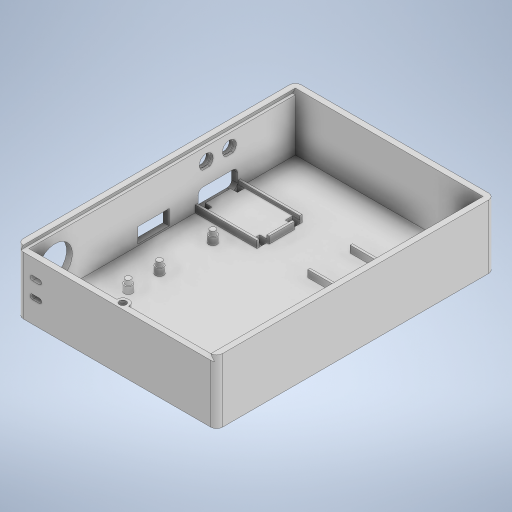
# Autodesk Inventor part: 01-Electronic-Compartment-Updated
Saved by Autodesk Inventor 2023 (Build 270158000, 158)
## iProperties
Created: 2024-02-14
Part Number: 01-Electronic-Compartment-Updated
Material: Generic
Document SubType Name: Modeling
Designer: ongyu
Density: 1 g/cm^3
Appearance: Default
Author: ongyu
Autodesk Inventor part; units mm, degrees
ref_plane "YZ Plane" through (0, 0, 0) normal (1, 0, 0) x (0, 1, 0)
ref_plane "XZ Plane" through (0, 0, 0) normal (0, 1, 0) x (-1, 0, 0)
sketch "Sketch1" plane through (0, 0, 0) normal (0, 1, 0) x (-1, 0, 0)
  line L0 (38, -43.8749) -> (-38, -43.8749)
  line L1 (-38, -43.8749) -> (-38, -23.8749)
  line L2 (-38, -23.8749) -> (38, -23.8749)
  line L3 (38, -23.8749) -> (38, -43.8749)
  line L4 (0, -70.3716) -> (0, 97.6051) projected
  line L5 (43, -43.8749) -> (-38, -43.8749)
  line L6 (-38, -43.8749) -> (-38, 71.1084)
  line L7 (-38, 71.1084) -> (43, 71.1084)
  line L8 (43, 71.1084) -> (43, -43.8749)
  circle A0 centre (-29.9129, 6.6001) radius 1.275
  circle A1 centre (-29.9129, 29.6501) radius 1.275
  circle A2 centre (28.1371, 6.6001) radius 1.275
  circle A3 centre (28.1371, 29.6501) radius 1.275
  line L9 (45.5, -46.3749) -> (-40.5, -46.3749)
  line L10 (-40.5, -46.3749) -> (-40.5, 73.6084)
  line L11 (-40.5, 73.6084) -> (45.5, 73.6084)
  line L12 (45.5, 73.6084) -> (45.5, -46.3749)
  line L13 (43, -18.8749) -> (14.338, -18.8749)
  line L14 (43, -1.8749) -> (14.338, -1.8749)
  line L15 (43, -18.8749) -> (40, -18.8749)
  line L16 (40, -18.8749) -> (40, -15.8749)
  line L17 (40, -15.8749) -> (43, -15.8749)
  line L18 (43, -15.8749) -> (43, -18.8749)
  line L19 (43, -1.8749) -> (40, -1.8749)
  line L20 (40, -1.8749) -> (40, -4.8749)
  line L21 (40, -4.8749) -> (43, -4.8749)
  line L22 (43, -4.8749) -> (43, -1.8749)
  line L23 (19.338, -1.8749) -> (16.338, -1.8749)
  line L24 (16.338, -1.8749) -> (16.338, -4.8749)
  line L25 (16.338, -4.8749) -> (19.338, -4.8749)
  line L26 (19.338, -4.8749) -> (19.338, -1.8749)
  line L27 (19.338, -18.8749) -> (16.338, -18.8749)
  line L28 (16.338, -18.8749) -> (16.338, -15.8749)
  line L29 (16.338, -15.8749) -> (19.338, -15.8749)
  line L30 (19.338, -15.8749) -> (19.338, -18.8749)
  line L31 (32, 3.1251) -> (-33, 3.1251)
  line L32 (-33, 3.1251) -> (-33, 33.1251)
  line L33 (-33, 33.1251) -> (32, 33.1251)
  line L34 (32, 33.1251) -> (32, 3.1251)
  line L35 (32, 18.1251) -> (-33, 18.1251)
  point P0 (0, 0)
  point P1 (43, -4.8749)
  point P2 (43, -15.8749)
  dimension "d0" = 76
  dimension "d1" = 20
  dimension "d2" = 38
  dimension "d4" = 5
  dimension "d5" = 0
  dimension "d14" = 2.55
  dimension "d15" = 2.55
  dimension "d17" = 2.55
  dimension "d18" = 58.05
  dimension "d24" = 81
  dimension "d31" = 0
  dimension "d32" = 2.5
  dimension "d33" = 2.5
  dimension "d34" = 2.5
  dimension "d35" = 2.5
  dimension "d72" = 17
  dimension "d73" = 28.662
  dimension "d74" = 28.662
  dimension "d75" = 3
  dimension "d76" = 3
  dimension "d77" = 3
  dimension "d78" = 3
  dimension "d79" = 2
  dimension "d80" = 3
  dimension "d81" = 3
  dimension "d82" = 3
  dimension "d83" = 3
  dimension "d115" = 65
  dimension "d116" = 30
  dimension "d119" = 5
  dimension "d120" = 5
  dimension "d209" = 114.9833
  dimension "d210" = 119.9833
  dimension "d268" = 5
  dimension "d270" = 3.0871
  dimension "d273" = 0
  dimension "d274" = 0
  dimension "d275" = 23.05
  dimension "d276" = 23.05
  constraints: 70 end point, 16 parallel, 10 horizontal, 9 perpendicular, 4 centre point, 4 point on line, 2 midpoint
  measures "d0" distance of L0.start L0.end
  measures "d1" distance of L2.end L0.start
  measures "d2" distance between parallel lines of L4 L3
  measures "d4" distance between parallel lines of L8 L3
  measures "d5" distance between parallel lines of L6 L1
  measures "d14" diameter of A0
  measures "d15" diameter of A1
  measures "d17" diameter of A2
  measures "d18" distance of A2.centre A0.centre
  measures "d24" distance of L5.start L5.end
  measures "d31" distance between parallel lines of L5 L0
  measures "d32" distance between parallel lines of L11 L7
  measures "d33" distance between parallel lines of L10 L6
  measures "d34" distance between parallel lines of L12 L8
  measures "d35" distance between parallel lines of L0 L9
  measures "d72" distance between parallel lines of L14 L13
  measures "d73" distance of L13.start L13.end
  measures "d74" distance of L14.start L14.end
  measures "d75" distance of L15.end L16.end
  measures "d76" distance of L16.end L17.end
  measures "d77" distance of L20.end L21.end
  measures "d78" distance of L19.end L20.end
  measures "d79" distance from line of L14.end L24
  measures "d80" distance of L24.end L25.end
  measures "d81" distance of L25.end L23.start
  measures "d82" distance of L28.end L29.end
  measures "d83" distance of L29.end L27.start
  measures "d115" distance between parallel lines of L34 L32
  measures "d116" distance between parallel lines of L33 L31
  measures "d119" distance between parallel lines of L13 L2
  measures "d120" distance between parallel lines of L31 L14
  measures "d209" distance between parallel lines of L7 L0
  measures "d210" distance between parallel lines of L11 L9
  measures "d268" distance between parallel lines of L6 L32
  measures "d270" distance from line of L32 A0.centre
  measures "d273" horizontal distance of A1.centre A0.centre
  measures "d274" horizontal distance of A3.centre A2.centre
  measures "d275" distance of A1.centre A0.centre
  measures "d276" distance of A2.centre A3.centre
extrude "Extrusion3" add sketch "Sketch1" along normal blind 25 contours L5 L8 L7 L4 L11 L12 L9 L0 | L4 L9 L10 L11 L7 L6 L1 L0
extrude "Extrusion12" add sketch "Sketch1" against normal blind 2.5 contours L5 L8 L7 L4 L11 L12 L9 L0 | L0 L4 L2 L3 | L3 L2 L4 L31 L34 L33 L7 L8 L14 L20 L21 L17 L16 L13 L5 | L4 L9 L10 L11 L7 L6 L1 L0 | L0 L1 L2 L4 | L2 L6 L7 L4 L33 L32 L31 | L13 L16 L17 L8 | L31 L32 L35 L4 | L4 L35 L34 L31 | L35 L32 L33 L4 | L4 L33 L34 L35 | L21 L20 L14 L8 | A0 | A1 | A2 | A3 | L13 L28 L29 L30 | L26 L25 L24 L14
fillet "Fillet6" radius 2.5 4 edges at (40.5, 11.25, 73.6084) (-45.5, 11.25, 73.6084) (40.5, 11.25, -46.3749) (-45.5, 11.25, -46.3749)
extrude "Extrusion1" add sketch "Sketch1" along normal blind 5 contours A0 | A2 | A3
sketch "Sketch11" plane through (0, 0, 0) normal (0, 1, 0) x (1, 0, 0)
  circle A0 centre (-28.1371, -6.6001) radius 1.275 projected
  circle A1 centre (-28.1371, -29.6501) radius 1.275 projected
  circle A2 centre (29.9129, -6.6001) radius 1.275 projected
  circle A3 centre (-28.1371, -6.6001) radius 1.775
  circle A4 centre (-28.1371, -29.6501) radius 1.775
  circle A5 centre (29.9129, -6.6001) radius 1.775
  point P0 (0, 0)
  point P1 (26.525, -36.3729)
  dimension "d105" = 3.55
  dimension "d107" = 3.55
  dimension "d108" = 3.55
  dimension "d109" = 2.55
  constraints: 3 centre point, 3 coincident
  measures "d105" diameter of A5
  measures "d107" diameter of A4
  measures "d108" diameter of A3
  measures "d109" diameter of A2
extrude "Extrusion13" add sketch "Sketch11" along normal blind 3 contours A0 | A1 | A2 | A3 | A4 | A5
extrude "Extrusion14" cut sketch "Sketch1" against normal blind 2 contours L13 L16 L17 L8 | L21 L20 L14 L8 | L13 L28 L29 L30 | L26 L25 L24 L14
sketch "Sketch12" plane through (-45.5, -2.5, -43.8749) normal (-1, 0, 0) x (0, 0, 1)
  line L0 (25, 2.5) -> (25, 0.5) projected
  line L1 (27, 2.5) -> (40, 2.5)
  line L2 (42, 4.5) -> (42, 8.5)
  line L3 (40, 10.5) -> (27, 10.5)
  line L4 (25, 8.5) -> (25, 4.5)
  arc A0 (27, 10.5) -> (25, 8.5) centre (27, 8.5) ccw
  arc A1 (25, 4.5) -> (27, 2.5) centre (27, 4.5) ccw
  arc A2 (40, 2.5) -> (42, 4.5) centre (40, 4.5) ccw
  arc A3 (42, 8.5) -> (40, 10.5) centre (40, 8.5) ccw
  point P0 (43.8749, 2.5)
  point P1 (42, 2.5)
  dimension "d124" = 8
  dimension "d125" = 2
  constraints: 8 end point, 8 point on circle, 8 tangent, 4 centre point, 3 equal radius, 2 parallel, 2 point on line, 1 horizontal, 1 perpendicular
  measures "d124" distance between parallel lines of L1 L3
  measures "d125" radius of A0
extrude "Extrusion15" cut sketch "Sketch12" against normal up to surface (2.5 mm away)
ref_plane "Work Plane6" through (-45.5, 2, -10.3749) normal (0, 0, 1) x (1, 0, 0)
sketch "Sketch13" plane through (-45.5, -2.5, -43.8749) normal (-1, 0, 0) x (0, 0, 1)
  circle A0 centre (28.5, 19.3463) radius 2.5
  circle A1 centre (38.5, 19.3463) radius 2.5
  line L0 (33.5, 33) -> (33.5, -5.5) projected
  point P0 (43.8749, 2.5)
  dimension "d128" = 5
  dimension "d129" = 5
  dimension "d130" = 5
  dimension "d131" = 5
  constraints: 2 centre point
  measures "d128" diameter of A0
  measures "d129" diameter of A1
  measures "d130" distance from line of L0 A0.centre
  measures "d131" distance from line of A1.centre L0
sketch "Sketch14" plane through (-43, 25, 71.1084) normal (1, 0, 0) x (0, 0, -1)
  circle A0 centre (86.4833, -8.1537) radius 2.5 projected
  circle A1 centre (76.4833, -8.1537) radius 2.5 projected
  arc A2 (78.1416, -10.6537) -> (74.825, -10.6537) centre (76.4833, -8.1537) ccw
  arc A3 (88.1416, -10.6537) -> (84.825, -10.6537) centre (86.4833, -8.1537) ccw
  line L0 (74.825, -10.6537) -> (78.1416, -10.6537)
  line L1 (84.825, -10.6537) -> (88.1416, -10.6537)
  point P0 (71.1084, -25)
  dimension "d132" = 6
  dimension "d133" = 6
  constraints: 4 end point, 4 point on circle, 2 centre point, 2 coincident, 2 horizontal, 2 tangent
  measures "d132" diameter of A3
  measures "d133" diameter of A2
sketch "Sketch15" plane through (-43, -2.5, 73.6084) normal (0, 0, 1) x (1, 0, 0)
  line L0 (3, 18.25) -> (8, 18.25)
  line L1 (8, 18.25) -> (8, 16.25)
  line L2 (8, 16.25) -> (3, 16.25)
  line L3 (3, 16.25) -> (3, 18.25)
  line L4 (3, 11.25) -> (8, 11.25)
  line L5 (8, 11.25) -> (8, 9.25)
  line L6 (8, 9.25) -> (3, 9.25)
  line L7 (3, 9.25) -> (3, 11.25)
  line L8 (0, 27.5) -> (81, 27.5) projected
  line L9 (0, 0) -> (0, 27.5) projected
  line L10 (81, 0) -> (0, 0) projected
  point P0 (43, 2.5)
  dimension "d138" = 5
  dimension "d139" = 2
  dimension "d140" = 2
  dimension "d141" = 5
  dimension "d143" = 5
  dimension "d144" = 3
  dimension "d174" = 27.5
  dimension "d175" = 9
  dimension "d176" = 9.25
  constraints: 16 end point, 4 parallel, 2 horizontal, 2 perpendicular, 1 point on line
  measures "d138" distance of L1.end L2.end
  measures "d139" distance of L0.end L1.end
  measures "d140" distance between parallel lines of L6 L4
  measures "d141" distance between parallel lines of L5 L7
  measures "d143" distance between parallel lines of L4 L2
  measures "d144" distance between parallel lines of L9 L3
  measures "d174" distance between parallel lines of L10 L8
  measures "d175" distance between parallel lines of L6 L0
  measures "d176" distance between parallel lines of L0 L8
extrude "Extrusion18" cut sketch "Sketch15" against normal up to surface (2.5 mm away)
sketch "Sketch16" plane through (-43, -2.5, 73.6084) normal (0, 0, 1) x (1, 0, 0)
  point P0 (43, 2.5)
fillet "Fillet7" radius 1 8 edges at (-40, 6.75, 72.3584) (-40, 13.75, 72.3584) (-40, 8.75, 72.3584) (-40, 15.75, 72.3584) (-35, 6.75, 72.3584) (-35, 8.75, 72.3584) (-35, 13.75, 72.3584) (-35, 15.75, 72.3584)
sketch "Sketch17" plane through (-45.5, -2.5, -43.8749) normal (-1, 0, 0) x (0, 0, 1)
  point P0 (43.8749, 2.5)
sketch "Sketch18" plane through (-45.5, -2.5, -43.8749) normal (-1, 0, 0) x (0, 0, 1)
  line L0 (54.5, 3.25) -> (68, 3.25)
  line L1 (68, 3.25) -> (68, 9.75)
  line L2 (68, 9.75) -> (54.5, 9.75)
  line L3 (54.5, 9.75) -> (54.5, 3.25)
  line L4 (40, 2.5) -> (27, 2.5) projected
  line L5 (27, 10.5) -> (40, 10.5) projected
  line L6 (0, 0) -> (0, 27.5) projected
  line L7 (25, 4.5) -> (25, 8.5) projected
  line L8 (114.9833, 0) -> (0, 0) projected
  line L9 (42, 8.5) -> (42, 4.5) projected
  point P0 (43.8749, 2.5)
  point P1 (42, 6.5)
  point P2 (54.5, 6.5)
  dimension "d150" = 6.5
  dimension "d151" = 13.5
  dimension "d152" = 8
  dimension "d195" = 2.5
  dimension "d196" = 0.75
  dimension "d261" = 12.5
  constraints: 8 end point, 2 midpoint, 2 parallel, 1 horizontal, 1 perpendicular
  measures "d150" distance between parallel lines of L0 L2
  measures "d151" distance between parallel lines of L3 L1
  measures "d152" distance between parallel lines of L4 L5
  measures "d195" distance between parallel lines of L8 L4
  measures "d196" distance between parallel lines of L5 L2
  measures "d261" distance of point (42, 6.5) point (54.5, 6.5)
extrude "Extrusion19" cut sketch "Sketch18" against normal up to surface (2.5 mm away)
sketch "Sketch19" plane through (-45.5, -2.5, -43.8749) normal (-1, 0, 0) x (0, 0, 1)
  line L0 (68, 9.75) -> (68, 3.25) projected
  line L1 (54.5, 3.25) -> (54.5, 9.75) projected
  line L2 (54.5, 9.75) -> (68, 9.75) projected
  line L3 (54.044, 16.1336) -> (68.456, 16.1336) construction
  line L4 (68.456, 16.1336) -> (68.456, 12.9572) construction
  line L5 (68.456, 12.9572) -> (54.044, 12.9572) construction
  line L6 (54.044, 12.9572) -> (54.044, 16.1336) construction
  spline S0 degree 2 poles (56.5091, 15.7211) (56.682, 15.5186) (56.8746, 14.9258) (56.8746, 14.5454) knots 0 0 0 1 2 2 2
  spline S1 degree 2 poles (56.8746, 14.5454) (56.8746, 14.1749) (56.6869, 13.5747) (56.5091, 13.3722) knots 0 0 0 1 2 2 2
  spline S2 degree 2 poles (56.5091, 13.3722) (56.3214, 13.1597) (55.8249, 12.9572) (55.526, 12.9572) knots 0 0 0 1 2 2 2
  spline S3 degree 2 poles (55.526, 12.9572) (55.2173, 12.9572) (54.7233, 13.1672) (54.5429, 13.3722) knots 0 0 0 1 2 2 2
  spline S4 degree 2 poles (54.5429, 13.3722) (54.3676, 13.5747) (54.1799, 14.17) (54.1799, 14.5454) knots 0 0 0 1 2 2 2
  spline S5 degree 2 poles (54.1799, 14.5454) (54.1799, 14.9283) (54.37, 15.5112) (54.5454, 15.7211) knots 0 0 0 1 2 2 2
  spline S6 degree 2 poles (54.5454, 15.7211) (54.7233, 15.9237) (55.2197, 16.1336) (55.526, 16.1336) knots 0 0 0 1 2 2 2
  spline S7 degree 2 poles (55.526, 16.1336) (55.8372, 16.1336) (56.3362, 15.9163) (56.5091, 15.7211) knots 0 0 0 1 2 2 2
  spline S8 degree 2 poles (56.4523, 14.5454) (56.4523, 14.8468) (56.3214, 15.3136) (56.2028, 15.4667) knots 0 0 0 1 2 2 2
  spline S9 degree 2 poles (56.2028, 15.4667) (56.0818, 15.6248) (55.7409, 15.7829) (55.5285, 15.7829) knots 0 0 0 1 2 2 2
  spline S10 degree 2 poles (55.5285, 15.7829) (55.3086, 15.7829) (54.9777, 15.6298) (54.8517, 15.4667) knots 0 0 0 1 2 2 2
  spline S11 degree 2 poles (54.8517, 15.4667) (54.7307, 15.3111) (54.6022, 14.8418) (54.6022, 14.5454) knots 0 0 0 1 2 2 2
  spline S12 degree 2 poles (54.6022, 14.5454) (54.6022, 13.9452) (55.1061, 13.3079) (55.5285, 13.3079) knots 0 0 0 1 2 2 2
  spline S13 degree 2 poles (55.5285, 13.3079) (55.9509, 13.3079) (56.4523, 13.9452) (56.4523, 14.5454) knots 0 0 0 1 2 2 2
  line L7 (59.5003, 13.0214) -> (59.0458, 13.0214)
  line L8 (59.0458, 13.0214) -> (57.6972, 15.6495)
  line L9 (57.6972, 15.6495) -> (57.6972, 13.0214)
  line L10 (57.6972, 13.0214) -> (57.3192, 13.0214)
  line L11 (57.3192, 13.0214) -> (57.3192, 16.0694)
  line L12 (57.3192, 16.0694) -> (57.8948, 16.0694)
  line L13 (57.8948, 16.0694) -> (59.1224, 13.6562)
  line L14 (59.1224, 13.6562) -> (59.1224, 16.0694)
  line L15 (59.1224, 16.0694) -> (59.5003, 16.0694)
  line L16 (59.5003, 16.0694) -> (59.5003, 13.0214)
  spline S14 degree 2 poles (63.5832, 15.7211) (63.7561, 15.5186) (63.9488, 14.9258) (63.9488, 14.5454) knots 0 0 0 1 2 2 2
  spline S15 degree 2 poles (63.9488, 14.5454) (63.9488, 14.1749) (63.761, 13.5747) (63.5832, 13.3722) knots 0 0 0 1 2 2 2
  spline S16 degree 2 poles (63.5832, 13.3722) (63.3955, 13.1597) (62.899, 12.9572) (62.6001, 12.9572) knots 0 0 0 1 2 2 2
  spline S17 degree 2 poles (62.6001, 12.9572) (62.2914, 12.9572) (61.7974, 13.1672) (61.6171, 13.3722) knots 0 0 0 1 2 2 2
  spline S18 degree 2 poles (61.6171, 13.3722) (61.4417, 13.5747) (61.254, 14.17) (61.254, 14.5454) knots 0 0 0 1 2 2 2
  spline S19 degree 2 poles (61.254, 14.5454) (61.254, 14.9283) (61.4442, 15.5112) (61.6195, 15.7211) knots 0 0 0 1 2 2 2
  spline S20 degree 2 poles (61.6195, 15.7211) (61.7974, 15.9237) (62.2939, 16.1336) (62.6001, 16.1336) knots 0 0 0 1 2 2 2
  spline S21 degree 2 poles (62.6001, 16.1336) (62.9114, 16.1336) (63.4103, 15.9163) (63.5832, 15.7211) knots 0 0 0 1 2 2 2
  spline S22 degree 2 poles (63.5264, 14.5454) (63.5264, 14.8468) (63.3955, 15.3136) (63.2769, 15.4667) knots 0 0 0 1 2 2 2
  spline S23 degree 2 poles (63.2769, 15.4667) (63.1559, 15.6248) (62.815, 15.7829) (62.6026, 15.7829) knots 0 0 0 1 2 2 2
  spline S24 degree 2 poles (62.6026, 15.7829) (62.3828, 15.7829) (62.0518, 15.6298) (61.9258, 15.4667) knots 0 0 0 1 2 2 2
  spline S25 degree 2 poles (61.9258, 15.4667) (61.8048, 15.3111) (61.6764, 14.8418) (61.6764, 14.5454) knots 0 0 0 1 2 2 2
  spline S26 degree 2 poles (61.6764, 14.5454) (61.6764, 13.9452) (62.1802, 13.3079) (62.6026, 13.3079) knots 0 0 0 1 2 2 2
  spline S27 degree 2 poles (62.6026, 13.3079) (63.025, 13.3079) (63.5264, 13.9452) (63.5264, 14.5454) knots 0 0 0 1 2 2 2
  line L17 (66.2162, 15.7088) -> (64.7985, 15.7088)
  line L18 (64.7985, 15.7088) -> (64.7985, 14.8492)
  line L19 (64.7985, 14.8492) -> (66.157, 14.8492)
  line L20 (66.157, 14.8492) -> (66.157, 14.4886)
  line L21 (66.157, 14.4886) -> (64.7985, 14.4886)
  line L22 (64.7985, 14.4886) -> (64.7985, 13.0214)
  line L23 (64.7985, 13.0214) -> (64.3934, 13.0214)
  line L24 (64.3934, 13.0214) -> (64.3934, 16.0694)
  line L25 (64.3934, 16.0694) -> (66.2162, 16.0694)
  line L26 (66.2162, 16.0694) -> (66.2162, 15.7088)
  line L27 (68.4022, 15.7088) -> (66.9844, 15.7088)
  line L28 (66.9844, 15.7088) -> (66.9844, 14.8492)
  line L29 (66.9844, 14.8492) -> (68.3429, 14.8492)
  line L30 (68.3429, 14.8492) -> (68.3429, 14.4886)
  line L31 (68.3429, 14.4886) -> (66.9844, 14.4886)
  line L32 (66.9844, 14.4886) -> (66.9844, 13.0214)
  line L33 (66.9844, 13.0214) -> (66.5793, 13.0214)
  line L34 (66.5793, 13.0214) -> (66.5793, 16.0694)
  line L35 (66.5793, 16.0694) -> (68.4022, 16.0694)
  line L36 (68.4022, 16.0694) -> (68.4022, 15.7088)
  point P0 (43.8749, 2.5)
  dimension "d160" = 13.5
  dimension "d263" = 0.456
  dimension "d264" = 0.456
  constraints: 2 other
  measures "d160" distance between parallel lines of L0 L1
  measures "d263" distance between parallel lines of L1 L6
  measures "d264" distance between parallel lines of L4 L0
sketch "Sketch20" plane through (-45.5, -2.5, -43.8749) normal (-1, 0, 0) x (0, 0, 1)
  circle A0 centre (103.7333, 13.75) radius 7.5
  line L0 (117.4833, 0) -> (117.4833, 27.5) projected
  line L1 (114.9833, 0) -> (0, 0) projected
  line L2 (0, 27.5) -> (114.9833, 27.5) projected
  point P0 (43.8749, 2.5)
  dimension "d166" = 15
  dimension "d167" = 13.75
  dimension "d168" = 13.75
  dimension "d172" = 27.5
  constraints: 1 centre point
  measures "d166" diameter of A0
  measures "d167" distance from line of L0 A0.centre
  measures "d168" distance from line of L1 A0.centre
  measures "d172" distance between parallel lines of L1 L2
extrude "Extrusion21" cut sketch "Sketch20" against normal up to surface (2.5 mm away)
sketch "Sketch21" plane through (-43, -2.5, 73.6084) normal (0, 0, 1) x (1, 0, 0)
  line L0 (0, 27.5) -> (0, 0) projected
  line L1 (81, 2.5) -> (81, 27.5) projected
  line L2 (0, 27.5) -> (81, 27.5)
  line L3 (-1.25, 25) -> (82.25, 25)
  line L4 (81, 0) -> (0, 0) projected
  line L5 (81, 2.5) -> (0, 2.5) projected
  line L6 (-1.25, 25) -> (0, 27.5)
  line L7 (81, 27.5) -> (82.25, 25)
  point P0 (43, 2.5)
  dimension "d180" = 2.5
  dimension "d181" = 2.5
  dimension "d182" = 1.25
  dimension "d183" = 1.25
  constraints: 8 end point, 2 horizontal, 1 parallel
  measures "d180" distance between parallel lines of L3 L2
  measures "d181" distance between parallel lines of L4 L5
  measures "d182" distance from line of L0 L3.start
  measures "d183" distance from line of L1 L3.end
extrude "Extrusion22" cut sketch "Sketch21" against normal up to surface (117.4833 mm away) contours L2 L1 L3 L0 | L0 L3 L6 | L7 L3 L1
ref_plane "Work Plane8" through (-45.5, 2, -5.3749) normal (0, 0, 1) x (1, 0, 0)
sketch "Sketch22" plane through (-45.5, 2, -5.3749) normal (0, 0, 1) x (1, 0, 0)
  circle A0 centre (1.25, 13) radius 2.5
  line L0 (2.5, -4.5) -> (83.5, -4.5) projected
  line L1 (0, -4.5) -> (0, 23) projected
  line L2 (1.25, 15.5) -> (3.25, 15.5)
  line L3 (3.25, 15.5) -> (3.25, 10.5)
  line L4 (3.25, 10.5) -> (1.25, 10.5)
  line L5 (-1.25, 13) -> (3.75, 13)
  point P0 (45.5, -2)
  point P1 (0, 13)
  point P2 (3.25, 13)
  point P3 (3.25, 14.5)
  point P4 (0, 15.1651)
  dimension "d188" = 5
  dimension "d189" = 17.5
  dimension "d191" = 1.25
  dimension "d192" = 2
  constraints: 8 end point, 4 point on circle, 2 horizontal, 1 centre point, 1 tangent, 1 vertical
  measures "d188" diameter of A0
  measures "d189" distance from line of L0 A0.centre
  measures "d191" distance from line of L1 A0.centre
  measures "d192" distance of L2.start L2.end
sketch "Sketch24" plane through (0, 0, 0) normal (0, 1, 0) x (1, 0, 0)
  circle A0 centre (-28.1371, -43.1501) radius 1.275
  circle A1 centre (-28.1371, -43.1501) radius 1.775
  circle A2 centre (-28.1371, -29.6501) radius 1.775 projected
  line L0 (-43, -73.6084) -> (-43, 43.8749) projected
  circle A3 centre (-28.1371, -29.6501) radius 1.275 projected
  circle A4 centre (30.2829, -43.1501) radius 1.275
  circle A5 centre (30.2829, -43.1501) radius 1.775
  circle A6 centre (-28.1371, -6.6001) radius 1.775 projected
  circle A7 centre (29.9129, -6.6001) radius 1.775 projected
  circle A8 centre (30.2829, -63.4701) radius 1.775
  circle A9 centre (30.2829, -63.4701) radius 1.275
  circle A10 centre (-28.1371, -6.6001) radius 1.275 projected
  line L1 (38, 43.8749) -> (38, -73.6084) projected
  point P0 (0, 0)
  dimension "d197" = 2.55
  dimension "d198" = 13.5
  dimension "d199" = 3.55
  dimension "d200" = 14.8629
  dimension "d201" = 14.8629
  dimension "d202" = 36.55
  dimension "d203" = 36.55
  dimension "d204" = 2.55
  dimension "d205" = 3.55
  dimension "d208" = 54.5
  dimension "d211" = 2.55
  dimension "d212" = 3.55
  dimension "d213" = 20.32
  dimension "d214" = 23.05
  dimension "d215" = 7.7171
  dimension "d248" = 58.42
  constraints: 6 centre point, 3 coincident
  measures "d197" diameter of A0
  measures "d198" distance of A2.centre A1.centre
  measures "d199" diameter of A1
  measures "d200" distance from line of L0 A1.centre
  measures "d201" distance from line of L0 A3.centre
  measures "d202" distance of A6.centre A0.centre
  measures "d203" vertical distance of A5.centre A7.centre
  measures "d204" diameter of A4
  measures "d205" diameter of A5
  measures "d211" diameter of A9
  measures "d212" diameter of A8
  measures "d213" distance of A9.centre A4.centre
  measures "d214" distance between centres of A3 A10
  measures "d215" distance from line of L1 A4.centre
  measures "d248" distance of A0.centre A4.centre
extrude "Extrusion23" add sketch "Sketch24" along normal blind 5 contours A0 | A4 | A9
extrude "Extrusion24" add sketch "Sketch24" along normal blind 3 contours A1 | A5 | A8 | A9
sketch "Sketch25" plane through (0, 0, 0) normal (0, 1, 0) x (1, 0, 0)
  line L0 (-43, -71.1084) -> (38, -71.1084) projected
  line L1 (-5, -71.1084) -> (0, -71.1084)
  line L2 (0, -71.1084) -> (0, -70.6084)
  line L3 (-2, -68.6084) -> (-3, -68.6084)
  line L4 (-5, -70.6084) -> (-5, -71.1084)
  line L5 (0, 70.3716) -> (0, -97.6051) projected
  arc A0 (0, -70.6084) -> (-2, -68.6084) centre (-2, -70.6084) ccw
  arc A1 (-3, -68.6084) -> (-5, -70.6084) centre (-3, -70.6084) ccw
  line L6 (-43, -73.6084) -> (-43, 43.8749) projected
  line L7 (38, 43.8749) -> (38, -73.6084) projected
  point P0 (0, 0)
  point P1 (0, -68.6084)
  point P2 (-5, -68.6084)
  dimension "d221" = 5
  dimension "d222" = 2.5
  dimension "d224" = 0
  dimension "d225" = 2
  dimension "d252" = 38
  dimension "d253" = 38
  dimension "d254" = 81
  constraints: 8 end point, 4 point on circle, 4 point on line, 4 tangent, 2 centre point, 2 parallel, 1 equal radius, 1 horizontal, 1 perpendicular
  measures "d221" distance of point (0, -68.608) point (-5, -68.608)
  measures "d222" distance of point (-5, -68.608) L1.start
  measures "d224" distance between parallel lines of L0 L1
  measures "d225" radius of A0
  measures "d252" distance between parallel lines of L7 L2
  measures "d253" distance between parallel lines of L6 L4
  measures "d254" distance between parallel lines of L6 L7
extrude "Extrusion25" add sketch "Sketch25" along normal up to surface (22.5 mm away)
sketch "Sketch26" plane through (-43, 22.5, 73.6084) normal (0, 1, 0) x (1, 0, 0)
  line L0 (43, 2.5) -> (81, 2.5) projected
  circle A0 centre (40.5, 2.5) radius 1.5
  line L1 (38, 3) -> (38, 2.5) projected
  line L2 (43, 2.5) -> (43, 3) projected
  line L3 (81, 0) -> (0, 0) projected
  point P0 (43, 73.6084)
  point P1 (40.5, 0)
  dimension "d229" = 3
  dimension "d257" = 5
  dimension "d258" = 2.5
  dimension "d267" = 2.5
  constraints: 1 centre point, 1 coincident, 1 midpoint
  measures "d229" diameter of A0
  measures "d257" distance between parallel lines of L1 L2
  measures "d258" distance from line of L1 A0.centre
  measures "d267" distance of point (40.5, 0) A0.centre
extrude "Extrusion26" cut sketch "Sketch26" against normal up to surface (22.5 mm away)
extrude "Extrusion27" cut sketch "Sketch13" against normal up to surface (2.5 mm away)
extrude "Extrusion28" cut sketch "Sketch14" against normal blind 1 contours A0 | L1 A3 | A1 | L0 A2
sketch "Sketch27" plane through (0, 0, 0) normal (0, 1, 0) x (1, 0, 0)
  line L0 (-16.338, 18.8749) -> (-16.338, 15.8749) projected
  line L1 (-16.338, 18.8749) -> (-43, 18.8749)
  line L2 (-43, 18.8749) -> (-43, 1.8749)
  line L3 (-43, 1.8749) -> (-16.338, 1.8749)
  line L4 (-16.338, 1.8749) -> (-16.338, 18.8749)
  line L5 (-19.338, 15.8749) -> (-19.338, 18.8749) projected
  line L6 (-16.338, 15.8749) -> (-19.338, 15.8749) projected
  line L7 (-19.338, 4.8749) -> (-16.338, 4.8749) projected
  line L8 (-19.338, 1.8749) -> (-19.338, 4.8749) projected
  line L9 (-40, 4.8749) -> (-40, 1.8749) projected
  line L10 (-43, 4.8749) -> (-40, 4.8749) projected
  line L11 (-40, 15.8749) -> (-43, 15.8749) projected
  line L12 (-40, 18.8749) -> (-40, 15.8749) projected
  line L13 (-43, 18.8749) -> (-43, 43.8749) projected
  line L14 (-43, 18.8749) -> (-16.338, 18.8749)
  line L15 (-16.338, 18.8749) -> (-16.338, 19.1249)
  line L16 (-16.338, 19.1249) -> (-43, 19.1249)
  line L17 (-43, 19.1249) -> (-43, 18.8749)
  line L18 (-16.338, 1.8749) -> (-19.338, 1.8749) projected
  line L19 (-43, 43.8749) -> (-43, -71.1084) projected
  line L20 (-16.338, 1.8749) -> (-43, 1.8749)
  line L21 (-43, 1.8749) -> (-43, 1.6249)
  line L22 (-43, 1.6249) -> (-16.338, 1.6249)
  line L23 (-16.338, 1.6249) -> (-16.338, 1.8749)
  line L24 (-43, 19.1249) -> (-16.338, 19.1249)
  line L25 (-16.338, 19.1249) -> (-16.338, 20.1249)
  line L26 (-16.338, 20.1249) -> (-43, 20.1249)
  line L27 (-43, 20.1249) -> (-43, 19.1249)
  line L28 (-16.338, 1.6249) -> (-43, 1.6249)
  line L29 (-43, 1.6249) -> (-43, 0.6249)
  line L30 (-43, 0.6249) -> (-16.338, 0.6249)
  line L31 (-16.338, 0.6249) -> (-16.338, 1.6249)
  point P0 (0, 0)
  point P1 (-16.338, 15.8749)
  point P2 (-43, 19.1249)
  dimension "d287" = 0.25
  dimension "d288" = 0.25
  dimension "d289" = 0
  dimension "d290" = 1
  dimension "d291" = 1
  constraints: 40 end point, 10 parallel, 5 horizontal, 5 perpendicular, 3 other
  measures "d287" distance of L15.end L14.end
  measures "d288" distance between parallel lines of L20 L22
  measures "d289" distance between parallel lines of L0 L15
  measures "d290" distance between parallel lines of L30 L28
  measures "d291" distance between parallel lines of L24 L26
extrude "Extrusion29" add sketch "Sketch27" along normal blind 1.5 contours L1 L13 L16 L15 | L4 L7 L8 L3 L9 L10 L2 L11 L12 L1 L5 L6 | L23 L22 L19 L3
sketch "Sketch29" plane through (0, 0, 0) normal (0, 1, 0) x (1, 0, 0)
  line L0 (-16.338, 15.8749) -> (-15.338, 15.8749)
  line L1 (-15.338, 15.8749) -> (-15.338, 4.8749)
  line L2 (-15.338, 4.8749) -> (-16.338, 4.8749)
  line L3 (-16.338, 4.8749) -> (-16.338, 15.8749)
  line L4 (-19.338, 4.8749) -> (-16.338, 4.8749) projected
  point P0 (0, 0)
  dimension "d240" = 1
  constraints: 8 end point, 2 parallel, 1 collinear, 1 horizontal, 1 perpendicular
  measures "d240" distance between parallel lines of L3 L1
extrude "Extrusion30" add sketch "Sketch29" along normal blind 3
sketch "Sketch33" plane through (38, 0, -43.8749) normal (-1, 0, 0) x (0, 0, 1)
  line L0 (0, 0) -> (21, 0)
  line L1 (21, 0) -> (21, 22.5)
  line L2 (114.9833, 22.5) -> (0, 22.5) projected
  line L3 (0, 0) -> (0, 22.5) projected
  point P0 (43.8749, 0)
  dimension "d243" = 21
  dimension "d244" = 90
  constraints: 4 end point, 1 horizontal, 1 point on line
  measures "d243" distance of L0.start L0.end
  measures "d244" angle of L1 L0
extrude "Extrusion31" cut sketch "Sketch33" against normal blind 1
thread "Thread2" size "M3x0.5" class "6H" standard "ANSI Metric M Profile" length 9
extrude "Extrusion32" cut sketch "Sketch19" against normal blind 2
sketch "Sketch34" plane through (0, 0, 0) normal (0, 1, 0) x (1, 0, 0)
  line L0 (5.5, 19.0249) -> (25.5, 19.0249)
  line L1 (25.5, 19.0249) -> (25.5, 20.0249)
  line L2 (25.5, 20.0249) -> (5.5, 20.0249)
  line L3 (5.5, 20.0249) -> (5.5, 19.0249)
  line L4 (25.5, 1.7249) -> (5.5, 1.7249)
  line L5 (5.5, 1.7249) -> (5.5, 0.7249)
  line L6 (5.5, 0.7249) -> (25.5, 0.7249)
  line L7 (25.5, 0.7249) -> (25.5, 1.7249)
  line L8 (38, 43.8749) -> (38, -73.6084) projected
  line L9 (-40, 1.8749) -> (-19.338, 1.8749) projected
  line L10 (-19.338, 18.8749) -> (-40, 18.8749) projected
  point P0 (0, 0)
  point P1 (5.5, 19.5249)
  dimension "d277" = 17.3
  dimension "d278" = 20
  dimension "d279" = 20
  dimension "d280" = 1
  dimension "d281" = 1
  dimension "d282" = 12.5
  dimension "d283" = 0.15
  dimension "d284" = 17
  constraints: 16 end point, 4 parallel, 2 horizontal, 2 perpendicular, 1 midpoint, 1 point on line
  measures "d277" distance between parallel lines of L0 L4
  measures "d278" distance between parallel lines of L5 L7
  measures "d279" distance from line of point (5.5, 19.525) L1
  measures "d280" distance between parallel lines of L4 L6
  measures "d281" distance between parallel lines of L2 L0
  measures "d282" distance between parallel lines of L8 L7
  measures "d283" distance between parallel lines of L4 L9
  measures "d284" distance between parallel lines of L10 L9
extrude "Extrusion33" add sketch "Sketch34" along normal blind 3
sketch "Sketch35" plane through (0, 0, 0) normal (0, 1, 0) x (1, 0, 0)
  line L0 (-43, 1.6249) -> (-16.338, 1.6249) projected
  line L1 (-43, -73.6084) -> (-43, 43.8749) projected
  line L2 (-16.338, 19.1249) -> (-43, 19.1249) projected
  line L3 (-43, 19.1249) -> (-16.338, 19.1249) projected
  line L4 (-43, 19.1249) -> (-16.338, 19.1249)
  line L5 (-16.338, 19.1249) -> (-16.338, 20.1249)
  line L6 (-16.338, 20.1249) -> (-43, 20.1249)
  line L7 (-43, 20.1249) -> (-43, 19.1249)
  line L8 (-43, -71.1084) -> (-43, 1.6249) projected
  line L9 (-43, 1.6249) -> (-16.338, 1.6249)
  line L10 (-16.338, 1.6249) -> (-16.338, 0.6249)
  line L11 (-16.338, 0.6249) -> (-43, 0.6249)
  line L12 (-43, 0.6249) -> (-43, 1.6249)
  line L13 (-16.338, 1.6249) -> (-16.338, 1.8749) projected
  line L14 (-16.338, 18.8749) -> (-16.338, 15.8749) projected
  point P0 (0, 0)
  point P1 (-43, 0.6249)
  point P2 (-16.338, 19.1249)
  dimension "d292" = 1
  dimension "d293" = 1
  dimension "d294" = 0
  dimension "d295" = 0
  constraints: 16 end point, 4 parallel, 2 horizontal, 2 perpendicular
  measures "d292" distance of L5.end L4.end
  measures "d293" distance between parallel lines of L11 L9
  measures "d294" distance between parallel lines of L13 L10
  measures "d295" distance between parallel lines of L14 L5
extrude "Extrusion34" add sketch "Sketch35" along normal blind 3
sketch "Sketch36" plane through (-45.5, -2.5, -43.8749) normal (-1, 0, 0) x (0, 0, 1)
  line L0 (55.4022, 17.0104) -> (55.6522, 17.0104)
  line L1 (55.6522, 17.0104) -> (55.6522, 11.7082)
  line L2 (55.6522, 11.7082) -> (55.4022, 11.7082)
  line L3 (55.4022, 11.7082) -> (55.4022, 17.0104)
  line L4 (62.4764, 16.7855) -> (62.7264, 16.7855)
  line L5 (62.7264, 16.7855) -> (62.7264, 11.419)
  line L6 (62.7264, 11.419) -> (62.4764, 11.419)
  line L7 (62.4764, 11.419) -> (62.4764, 16.7855)
  line L8 (66.2162, 16.0694) -> (66.2162, 15.7088) projected
  line L9 (66.2162, 15.7088) -> (64.7985, 15.7088) projected
  line L10 (64.7985, 15.7088) -> (64.7985, 14.8492) projected
  line L11 (64.7985, 14.8492) -> (66.157, 14.8492) projected
  line L12 (66.157, 14.8492) -> (66.157, 14.4886) projected
  line L13 (66.157, 14.4886) -> (64.7985, 14.4886) projected
  line L14 (64.7985, 14.4886) -> (64.7985, 13.0214) projected
  line L15 (64.7985, 13.0214) -> (64.3934, 13.0214) projected
  line L16 (64.3934, 13.0214) -> (64.3934, 16.0694) projected
  line L17 (64.3934, 16.0694) -> (66.2162, 16.0694) projected
  line L18 (59.5003, 16.0694) -> (59.5003, 13.0214) projected
  line L19 (59.5003, 13.0214) -> (59.0458, 13.0214) projected
  line L20 (59.0458, 13.0214) -> (57.6972, 15.6495) projected
  line L21 (57.6972, 15.6495) -> (57.6972, 13.0214) projected
  line L22 (57.6972, 13.0214) -> (57.3192, 13.0214) projected
  line L23 (57.3192, 13.0214) -> (57.3192, 16.0694) projected
  line L24 (57.3192, 16.0694) -> (57.8948, 16.0694) projected
  line L25 (57.8948, 16.0694) -> (59.1224, 13.6562) projected
  line L26 (59.1224, 13.6562) -> (59.1224, 16.0694) projected
  line L27 (59.1224, 16.0694) -> (59.5003, 16.0694) projected
  line L28 (68.4022, 16.0694) -> (68.4022, 15.7088) projected
  line L29 (68.4022, 15.7088) -> (66.9844, 15.7088) projected
  line L30 (66.9844, 15.7088) -> (66.9844, 14.8492) projected
  line L31 (66.9844, 14.8492) -> (68.3429, 14.8492) projected
  line L32 (68.3429, 14.8492) -> (68.3429, 14.4886) projected
  line L33 (68.3429, 14.4886) -> (66.9844, 14.4886) projected
  line L34 (66.9844, 14.4886) -> (66.9844, 13.0214) projected
  line L35 (66.9844, 13.0214) -> (66.5793, 13.0214) projected
  line L36 (66.5793, 13.0214) -> (66.5793, 16.0694) projected
  line L37 (66.5793, 16.0694) -> (68.4022, 16.0694) projected
  circle A0 centre (38.5, 19.3463) radius 2.5 projected
  circle A1 centre (28.5, 19.3463) radius 2.5 projected
  circle A2 centre (103.7333, 13.75) radius 7.5 projected
  line L38 (68, 3.25) -> (54.5, 3.25) projected
  line L39 (54.5, 3.25) -> (54.5, 9.75) projected
  line L40 (54.5, 9.75) -> (68, 9.75) projected
  line L41 (68, 9.75) -> (68, 3.25) projected
  line L42 (25, 4.5) -> (25, 8.5) projected
  arc A3 (27, 10.5) -> (25, 8.5) centre (27, 8.5) ccw projected
  line L43 (27, 10.5) -> (40, 10.5) projected
  arc A4 (42, 8.5) -> (40, 10.5) centre (40, 8.5) ccw projected
  line L44 (42, 8.5) -> (42, 4.5) projected
  arc A5 (40, 2.5) -> (42, 4.5) centre (40, 4.5) ccw projected
  line L45 (40, 2.5) -> (27, 2.5) projected
  arc A6 (25, 4.5) -> (27, 2.5) centre (27, 4.5) ccw projected
  line L46 (0, 0) -> (0, 27.5) projected
  line L47 (114.9833, 0) -> (0, 0) projected
  line L48 (114.9833, 27.5) -> (114.9833, 0) projected
  line L49 (0, 27.5) -> (114.9833, 27.5) projected
  point P0 (43.8749, 2.5)
  dimension "d298" = 0.25
  dimension "d299" = 2.6948
  dimension "d300" = 1.2224
  dimension "d302" = 2.6948
  dimension "d303" = 1.2224
  dimension "d304" = 0.25
  constraints: 16 end point, 4 parallel, 2 horizontal, 2 perpendicular, 17 other
  measures "d298" distance between parallel lines of L1 L3
  measures "d299" distance of point (56.875, 14.545) point (54.18, 14.545)
  measures "d300" distance from line of L1 point (56.875, 14.545)
  measures "d302" distance of point (63.949, 14.545) point (61.254, 14.545)
  measures "d303" distance from line of point (61.254, 14.545) L7
  measures "d304" distance between parallel lines of L5 L7
extrude "Extrusion35" add sketch "Sketch36" against normal up to surface (2 mm away) contours L0 L1 L2 L3 | L4 L5 L6 L7
equation "\"d2\" = 0.5 * d0"
equation "\"d15\" = d14"
equation "\"d17\" = d14"
equation "\"d33\" = d32"
equation "\"d34\" = d32"
equation "\"d35\" = d33"
equation "\"d74\" = d73"
equation "\"d76\" = d75"
equation "\"d77\" = d76"
equation "\"d78\" = d75"
equation "\"d80\" = d77"
equation "\"d81\" = d78"
equation "\"d82\" = d80"
equation "\"d83\" = d75"
equation "\"d107\" = d106"
equation "\"d108\" = d107"
equation "\"d106\" = d105"
body "Solid1"
